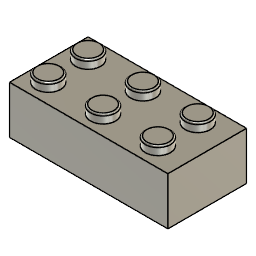
Day1-LegoBrick (Autodesk Fusion 360 design; units mm, degrees)
part number: 2025-11-17-19-23-03-980
Autodesk Fusion 360 part; units mm, degrees
sketch "Sketch1" plane through (0, 0, 0) normal (0, 0, 1) x (1, 0, 0)
  line L0 (0, 0) -> (31.8, 0)
  line L1 (31.8, 0) -> (31.8, 15.8)
  line L2 (31.8, 15.8) -> (0, 15.8)
  line L3 (0, 15.8) -> (0, 0)
  dimension "d1" = 31.8
  dimension "d2" = 15.8
  constraint horizontal L0
  constraint vertical L1
  constraint horizontal L2
  constraint vertical L3
  constraint coincident L0.start L3.end
  measures "d1" distance of L1 L3
  measures "d2" distance of L0 L2
extrude "Extrude1" add sketch "Sketch1" along normal blind 9.6 makes body 1
sketch "Sketch2" plane through (0, 0, 9.6) normal (0, 0, 1) x (-1, 0, 0)
  line L0 (0, -15.8) -> (0, 0)
  line L1 (0, 0) -> (-31.8, 0)
  line L2 (-31.8, 0) -> (-31.8, -15.8)
  line L3 (-31.8, -15.8) -> (0, -15.8)
  circle A0 centre (-3.9, -11.9) radius 2.5
  dimension "d5" = 5
  dimension "d6" = 3.9
  dimension "d7" = 3.9
  measures "d5" diameter of A0
  measures "d6" distance of L0 A0.centre
  measures "d7" distance of L3 A0.centre
extrude "Extrude2" add sketch "Sketch2" along normal blind 1.7 contours A0 bodies 1
pattern_linear "R-Pattern1" count 2 spacing 8 along (0, -1, 0) count 3 spacing 11 along (1, 0, 0) of "Extrude2"
shell "Shell1" thickness 1.49 removed faces 1 at (10.6, 10.5333, 0) on bodies 1
sketch "Sketch3" plane through (0, 0, 0) normal (0, 0, 1) x (1, 0, 0)
  circle A0 centre (9.5, 8) radius 3.15
  circle A1 centre (9.5, 8) radius 4.15
  dimension "d15" = 6.3
  dimension "d16" = 1
  measures "d15" diameter of A0
extrude "Extrude3" add sketch "Sketch3" along normal blind 8.1 separate body makes body 2
pattern_linear "R-Pattern2" count 1 spacing 0 along (0, -1, 0) count 2 spacing 11 along (1, 0, 0) of "Extrude3" makes body 3
fillet "Fillet1" radius 0.3 6 edges at (6.2308, 12.804, 11.3) (17.2308, 12.804, 11.3) (28.2308, 12.804, 11.3) (28.2308, 4.804, 11.3) (17.2308, 4.804, 11.3) (6.2308, 4.804, 11.3) on bodies 1
